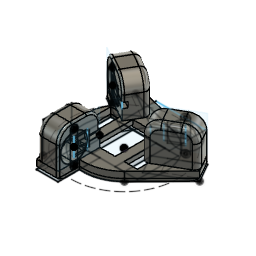
head (Autodesk Fusion 360 design; units mm, degrees)
Autodesk Fusion 360 part; units mm, degrees
note: some values were not read from the file. Set by a fixed rule: which sketch regions a step uses.
sketch "Sketch1" plane through (0, 0, 0) normal (0, 1, 0) x (1, 0, 0)
  line L0 (-38, 23) -> (38, 23)
  line L1 (38, 23) -> (38, -23)
  line L2 (38, -23) -> (-38, -23)
  line L3 (-38, -23) -> (-38, 23)
  line L4 (-28, 23) -> (28, 23)
  line L5 (28, 23) -> (28, 63.9462)
  line L6 (28, 63.9462) -> (-28, 63.9462)
  line L7 (-28, 63.9462) -> (-28, 23)
  circle A0 centre (0, 0) radius 60 construction
  line L8 (-4.5, -70) -> (-28.5, -70)
  line L9 (-28.5, -70) -> (-28.5, -23)
  line L10 (-28.5, -23) -> (-4.5, -23)
  line L11 (-4.5, -23) -> (-4.5, -70)
  line L12 (-4.5, -67) -> (-24.5, -67) construction
  line L13 (-24.5, -67) -> (-24.5, -37) construction
  line L14 (-24.5, -37) -> (-4.5, -37) construction
  line L15 (-4.5, -37) -> (-4.5, -67) construction
  line L16 (34.1686, -13.1817) -> (22.1686, 7.6029)
  line L17 (74.8718, 10.3183) -> (34.1686, -13.1817)
  line L18 (22.1686, 7.6029) -> (62.8718, 31.1029)
  line L19 (62.8718, 31.1029) -> (74.8718, 10.3183)
  line L20 (70.2737, 12.2824) -> (44.2929, -2.7176) construction
  line L21 (44.2929, -2.7176) -> (34.2929, 14.6029) construction
  line L22 (60.2737, 29.6029) -> (70.2737, 12.2824) construction
  line L23 (34.2929, 14.6029) -> (60.2737, 29.6029) construction
  line L24 (-5.6686, 36.1817) -> (-17.6686, 15.3971)
  line L25 (-46.3718, 59.6817) -> (-5.6686, 36.1817)
  line L26 (-17.6686, 15.3971) -> (-58.3718, 38.8971)
  line L27 (-58.3718, 38.8971) -> (-46.3718, 59.6817)
  line L28 (-45.7737, 54.7176) -> (-19.7929, 39.7176) construction
  line L29 (-19.7929, 39.7176) -> (-29.7929, 22.3971) construction
  line L30 (-55.7737, 37.3971) -> (-45.7737, 54.7176) construction
  line L31 (-29.7929, 22.3971) -> (-55.7737, 37.3971) construction
  circle A1 centre (0, 0) radius 46
  line L32 (-28.5, -70) -> (-44.3617, -12.167)
  line L33 (74.8718, 10.3183) -> (32.7178, -32.3349)
  line L34 (-46.3718, 59.6817) -> (11.6439, 44.5019)
  line L35 (-23, -23) -> (-13, -23)
  line L36 (-13, -23) -> (-13, 23)
  line L37 (-13, 23) -> (-23, 23)
  line L38 (-23, 23) -> (-23, -23)
  line L39 (13, -23) -> (23, -23)
  line L40 (23, -23) -> (23, 23)
  line L41 (23, 23) -> (13, 23)
  line L42 (13, 23) -> (13, -23)
  dimension "d1" = 76
  dimension "d2" = 38
  dimension "d3" = 46
  dimension "d4" = 23
  dimension "d5" = 56
  dimension "d6" = 28
  dimension "d7" = 120
  dimension "d8" = 24
  dimension "d9" = 4.5
  dimension "d10" = 70
  dimension "d11" = 20
  dimension "d12" = 30
  dimension "d13" = 67
  dimension "d15" = 360
  dimension "d16" = 92
  dimension "d18" = 360
  dimension "d24" = 15
  dimension "d25" = 10
  dimension "d26" = 10
  dimension "d27" = 15
  constraint horizontal L0
  constraint vertical L1
  constraint horizontal L2
  constraint vertical L3
  constraint horizontal L4
  constraint vertical L5
  constraint horizontal L6
  constraint vertical L7
  constraint coincident L0 L4.start
  constraint coincident A0.centre A1.centre
  constraint horizontal L8
  constraint vertical L9
  constraint horizontal L10
  constraint vertical L11
  constraint coincident L2 L9.end
  constraint horizontal L12
  constraint vertical L13
  constraint horizontal L14
  constraint vertical L15
  constraint coincident L11 L12.start
  constraint concentric A0 A1
  constraint coincident A1 L32.end
  constraint tangent A1 L32
  constraint horizontal L35
  constraint vertical L36
  constraint horizontal L37
  constraint vertical L38
  constraint coincident L0 L36.end
  constraint coincident L10 L35.start
  constraint horizontal L39
  constraint vertical L40
  constraint horizontal L41
  constraint vertical L42
  constraint coincident L0 L40.end
  constraint coincident L2 L39.start
  measures "d1" distance of L0.start L0.end
  measures "d2" distance of A0.centre L3
  measures "d3" distance of L0.start L2.end
  measures "d4" distance of A0.centre L0
  measures "d5" distance of L5.end L6.end
  measures "d6" distance of A0.centre L7
  measures "d7" diameter of A0
  measures "d8" distance of L8.start L8.end
  measures "d9" distance of A0.centre L11
  measures "d10" distance of A0.centre L8
  measures "d11" distance of L12.start L12.end
  measures "d12" distance of L12.start L14.end
  measures "d13" distance of A0.centre L12
  measures "d16" diameter of A1
  measures "d24" distance of L3 L38
  measures "d25" distance of L36 L38
  measures "d26" distance of L40 L42
  measures "d27" distance of L1 L40
extrude "Extrude1" add sketch "Sketch1" along normal blind 3 contours L0 L7 L26 A1 | L0 L2 L3 L9 L26 A1 | L7 L25 L26 L27 A1 | L2 L9 L10 L11 A1 L35 | L9 A1 L32 | L8 L9 L11 A1 | L0 L1 L5 L18 A1 | L1 L2 L11 L17 A1 L39 | L17 L18 L19 A1 | L17 A1 L33 makes body 1 at (-23.6667, 0, 46.2598)
extrude "Extrude2" add sketch "Sketch1" along normal blind 2 from surface at 3 separate body contours L0 L4 L7 L24 L25 A1 L37 | L0 L7 L26 A1 | L0 L2 L3 L9 L26 A1 | L7 L25 L26 L27 A1 | L7 L25 A1 | L0 L4 L5 L24 L25 A1 L37 L41 | L7 L25 L34 | L7 L25 A1 L34 | L2 L9 L10 L11 A1 L35 | L9 A1 L32 | L8 L9 L11 A1 | L0 L1 L5 L18 A1 | L1 L2 L11 L17 A1 L39 | L1 L17 L18 A1 | L17 L18 L19 A1 | L17 A1 L33 makes body 2
extrude "Extrude3" add sketch "Sketch1" along normal blind 5 from surface at 5 contours L0 L4 L7 L24 L25 A1 L37 | L0 L7 L26 A1 | L0 L4 L24 L26 L37 L38 | L0 L2 L3 L9 L26 A1 | L7 L25 L26 L27 A1 | L7 L25 A1 | L0 L4 L5 L24 L25 A1 L37 L41 | L0 L2 L4 L10 L24 L26 L35 L36 L37 L38 | L7 L25 L34 | L7 L25 A1 L34 | L2 L9 L10 L11 A1 L35 | L9 A1 L32 | L0 L2 L4 L16 L18 L39 L40 L41 L42 | L8 L9 L11 A1 | L0 L1 L5 L18 A1 | L1 L2 L11 L17 A1 L39 | L1 L17 L18 A1 | L17 L18 L19 A1 | L17 A1 L33 bodies 2
extrude "Extrude4" add sketch "Sketch1" along normal blind 40 from surface at 10 separate body contours L0 L4 L7 L24 L25 A1 L37 | L0 L4 L26 L38 | L0 L7 L26 A1 | L0 L4 L24 L26 L37 L38 | L7 L25 L26 L27 A1 | L7 L25 A1 | L2 L9 L10 L11 A1 L35 | L8 L9 L11 A1 | L1 L17 L18 A1 | L17 L18 L19 A1 | L16 L18 L40 | L1 L16 L17 L18 L40 makes body 3 at (61.304, 36.6667, -2.4849) makes body 4 at (-4.5, 36.6667, 38.6667) makes body 5 at (-32.804, 36.6667, -51.8484)
sketch "Sketch2" plane through (-4.5, 0, 0) normal (1, 0, 0) x (0, 0, -1)
  line L0 (-70, 10) -> (-23, 10)
  line L1 (-23, 10) -> (-23, 50)
  line L2 (-23, 50) -> (-70, 50)
  line L3 (-70, 50) -> (-70, 10)
  circle A0 centre (-52, 25) radius 15
  circle A1 centre (-52, 42.75) radius 4
  circle A2 centre (-52, 7.25) radius 4
  line L4 (-56, 42.75) -> (-56, 7.25)
  line L5 (-48, 42.75) -> (-48, 7.25)
  line L6 (-52, 33) -> (-35, 33)
  line L7 (-35, 33) -> (-35, 17)
  line L8 (-35, 17) -> (-52, 17)
  line L9 (-52, 17) -> (-52, 33)
  line L10 (-52, 28) -> (-23, 28)
  line L11 (-23, 28) -> (-23, 22)
  line L12 (-23, 22) -> (-52, 22)
  line L13 (-52, 22) -> (-52, 28)
  circle A3 centre (-52, 42.75) radius 1.3
  circle A4 centre (-52, 7.25) radius 1.3
  line L14 (-52, 35) -> (-37, 35)
  line L15 (-37, 35) -> (-37, 15)
  line L16 (-37, 15) -> (-52, 15)
  line L17 (-52, 15) -> (-52, 35)
  dimension "d34" = 30
  dimension "d35" = 18
  dimension "d36" = 8
  dimension "d37" = 8
  dimension "d38" = 35.5
  dimension "d39" = 17.75
  dimension "d40" = 16
  dimension "d41" = 8
  dimension "d42" = 17
  dimension "d43" = 6
  dimension "d44" = 3
  dimension "d45" = 2.6
  dimension "d46" = 2.6
  dimension "d47" = 20
  dimension "d48" = 10
  constraint vertical A0.centre A1.centre
  constraint vertical A0.centre A2.centre
  constraint tangent L0 A0
  constraint coincident A1 L4.start
  constraint coincident A2 L4.end
  constraint tangent A2 L4
  constraint coincident A1 L5.start
  constraint coincident A2 L5.end
  constraint perpendicular L0 L5
  constraint tangent A1 L5
  constraint tangent A1 L4
  constraint horizontal L6
  constraint vertical L7
  constraint horizontal L8
  constraint vertical L9
  constraint coincident A0.centre L9
  constraint horizontal L10
  constraint vertical L11
  constraint horizontal L12
  constraint vertical L13
  constraint coincident L1 L11.end
  constraint coincident L9 L10.start
  constraint concentric A1 A3
  constraint concentric A2 A4
  constraint horizontal L14
  constraint vertical L15
  constraint horizontal L16
  constraint vertical L17
  measures "d34" diameter of A0
  measures "d35" distance of L3 A0.centre
  measures "d36" diameter of A1
  measures "d37" diameter of A2
  measures "d38" distance of A1.centre A2.centre
  measures "d39" distance of A0.centre A2.centre
  measures "d40" distance of L6.end L7.end
  measures "d41" distance of A0.centre L8
  measures "d42" distance of A0.centre L7
  measures "d43" distance of L10.end L11.end
  measures "d44" distance of A0.centre L10
  measures "d45" diameter of A3
  measures "d46" diameter of A4
  measures "d47" distance of L14.end L15.end
  measures "d48" distance of A0.centre L14
extrude "Extrude5" cut sketch "Sketch2" against normal blind 20 contours A0 A1 A2 L4 L5 L9 L13 L14 L16 L17 | A0 L4 | A0 A2 | A0 A1 | L6 L7 L10 L15 | L7 L10 L12 L15 | A0 L5 L16 | L7 L8 L12 L15 | A0 L10 L15 | A0 L6 L10 L15 | A0 L5 L8 L16 | A0 L8 L15 L16 | L5 L8 L16 L17 | A0 L5 L14 | A0 L8 L12 L15 | A0 L12 L15 | A0 L6 L14 L15 | A0 L5 L6 L10 | A0 L5 L10 L12 | A0 L5 L8 L12 | L5 L8 L9 L12 L17 | A0 L5 L6 L14 | L5 L6 L14 L17 | L5 L6 L9 L10 L17 | L5 L9 L10 L12 L13 L17 | A3 | A4 picked at (-52, 39.5657) bodies 2 4
extrude "Extrude6" cut sketch "Sketch2" against normal blind 5 contours L1 L7 L10 L11 L12 bodies 4
extrude "Extrude7" cut sketch "Sketch2" against normal blind 1 contours L0 A0 A2 L4 | L0 A2 L4 | L0 A0 A2 | L0 A2 | L0 A0 A2 | A0 A1 L4 | L0 A2 L5 | L0 A0 A2 L5 | A0 A1 | A0 A1 L5 picked at (-53.5011, 40.5339) bodies 2 4
sketch "Sketch3" plane through (2.25, 0, -3.8971) normal (-0.5, 0, 0.866025) x (0.866025, 0, 0.5)
  line L0 (-70, 10) -> (-23, 10)
  line L1 (-23, 10) -> (-23, 50)
  line L2 (-23, 50) -> (-70, 50)
  line L3 (-70, 50) -> (-70, 10)
  circle A0 centre (-52, 25) radius 15
  circle A1 centre (-52, 42.75) radius 4
  circle A2 centre (-52, 7.25) radius 4
  line L4 (-52, 35) -> (-37, 35)
  line L5 (-37, 35) -> (-37, 15)
  line L6 (-37, 15) -> (-52, 15)
  line L7 (-52, 15) -> (-52, 35)
  line L8 (-52, 33) -> (-35, 33)
  line L9 (-35, 33) -> (-35, 17)
  line L10 (-35, 17) -> (-52, 17)
  line L11 (-52, 17) -> (-52, 33)
  line L12 (-52, 28) -> (-23, 28)
  line L13 (-23, 28) -> (-23, 22)
  line L14 (-23, 22) -> (-52, 22)
  line L15 (-52, 22) -> (-52, 28)
  line L16 (-56, 42.75) -> (-56, 7.25)
  line L17 (-48, 7.25) -> (-48, 42.75)
  circle A3 centre (-52, 42.75) radius 1.3
  circle A4 centre (-52, 7.25) radius 1.3
  dimension "d55" = 30
  dimension "d56" = 8
  dimension "d57" = 8
  dimension "d58" = 18
  dimension "d59" = 35.5
  dimension "d60" = 17.75
  dimension "d61" = 6
  dimension "d62" = 16
  dimension "d63" = 20
  dimension "d64" = 10
  dimension "d65" = 8
  dimension "d66" = 3
  dimension "d67" = 17
  dimension "d68" = 2.6
  dimension "d69" = 2.6
  constraint vertical A0.centre A2.centre
  constraint vertical A0.centre A1.centre
  constraint tangent L0 A0
  constraint horizontal L4
  constraint vertical L5
  constraint horizontal L6
  constraint vertical L7
  constraint horizontal L8
  constraint vertical L9
  constraint horizontal L10
  constraint vertical L11
  constraint coincident L7 L8.start
  constraint horizontal L12
  constraint vertical L13
  constraint horizontal L14
  constraint vertical L15
  constraint coincident L7 L12.start
  constraint tangent A0 L5
  constraint coincident A0.centre L7
  constraint coincident A1 L16.start
  constraint coincident A2 L16.end
  constraint perpendicular L0 L16
  constraint coincident A2 L17.start
  constraint coincident A1 L17.end
  constraint tangent A1 L17
  constraint tangent A1 L16
  constraint tangent A2 L17
  constraint concentric A1 A3
  constraint concentric A2 A4
  measures "d55" diameter of A0
  measures "d56" diameter of A1
  measures "d57" diameter of A2
  measures "d58" distance of L3 A0.centre
  measures "d59" distance of A1.centre A2.centre
  measures "d60" distance of A0.centre A2.centre
  measures "d61" distance of L12.end L13.end
  measures "d62" distance of L8.end L9.end
  measures "d63" distance of L4.end L5.end
  measures "d64" distance of A0.centre L4
  measures "d65" distance of A0.centre L8
  measures "d66" distance of A0.centre L12
  measures "d67" distance of L8.start L8.end
  measures "d68" diameter of A3
  measures "d69" diameter of A4
extrude "Extrude8" cut sketch "Sketch3" against normal blind 20 contours A0 A1 A2 L4 L6 L7 L11 L15 L16 L17 | A0 L16 | A0 A2 | A0 A1 | L5 L8 L9 L12 | L5 L9 L12 L14 | A0 L6 L17 | L5 L9 L10 L14 | A0 L5 L8 L12 | A0 L5 L12 | A0 L6 L10 L17 | A0 L5 L6 L10 | L6 L7 L10 L17 | A0 L4 L17 | A0 L5 L14 | A0 L5 L10 L14 | A0 L4 L5 L8 | A0 L12 L14 L17 | A0 L8 L12 L17 | A0 L10 L14 L17 | L7 L10 L11 L14 L17 | A0 L4 L8 L17 | L4 L7 L8 L17 | L7 L11 L12 L14 L15 L17 | L7 L8 L11 L12 L17 | A3 | A4 picked at (-52, 39.5657) bodies 2 5
extrude "Extrude9" cut sketch "Sketch3" against normal blind 5 contours L1 L9 L12 L13 L14 bodies 5
extrude "Extrude10" cut sketch "Sketch3" against normal blind 1 contours L0 A0 A2 L16 | L0 A2 L16 | L0 A0 A2 | L0 A2 | L0 A0 A2 | A0 A1 L16 | L0 A2 L17 | L0 A0 A2 L17 | A0 A1 | A0 A1 L17 picked at (-50.4989, 40.5339) bodies 2 5
sketch "Sketch4" plane through (2.25, 0, 3.8971) normal (-0.5, 0, -0.866025) x (-0.866025, 0, 0.5)
  line L0 (-70, 10) -> (-23, 10)
  line L1 (-23, 10) -> (-23, 50)
  line L2 (-23, 50) -> (-70, 50)
  line L3 (-70, 50) -> (-70, 10)
  circle A0 centre (-52, 25) radius 15
  circle A1 centre (-52, 42.75) radius 4
  circle A2 centre (-52, 7.25) radius 4
  circle A3 centre (-52, 42.75) radius 1.3
  circle A4 centre (-52, 7.25) radius 1.3
  line L4 (-56, 7.25) -> (-56, 42.75)
  line L5 (-48, 42.75) -> (-48, 7.25)
  line L6 (-52, 35) -> (-37, 35)
  line L7 (-37, 35) -> (-37, 15)
  line L8 (-37, 15) -> (-52, 15)
  line L9 (-52, 15) -> (-52, 35)
  line L10 (-52, 33) -> (-34, 33)
  line L11 (-34, 33) -> (-34, 17)
  line L12 (-34, 17) -> (-52, 17)
  line L13 (-52, 17) -> (-52, 33)
  line L14 (-52, 28) -> (-23, 28)
  line L15 (-23, 28) -> (-23, 22)
  line L16 (-23, 22) -> (-52, 22)
  line L17 (-52, 22) -> (-52, 28)
  dimension "d76" = 30
  dimension "d77" = 8
  dimension "d78" = 8
  dimension "d79" = 17.75
  dimension "d80" = 35.5
  dimension "d81" = 18
  dimension "d82" = 2.6
  dimension "d83" = 2.6
  dimension "d84" = 20
  dimension "d85" = 10
  dimension "d86" = 16
  dimension "d87" = 8
  dimension "d88" = 3
  dimension "d89" = 6
  constraint vertical A0.centre A2.centre
  constraint vertical A0.centre A1.centre
  constraint concentric A1 A3
  constraint concentric A2 A4
  constraint tangent L0 A0
  constraint coincident A2 L4.start
  constraint coincident A1 L4.end
  constraint tangent A1 L4
  constraint coincident A1 L5.start
  constraint coincident A2 L5.end
  constraint tangent A2 L5
  constraint tangent A2 L4
  constraint tangent A1 L5
  constraint horizontal L6
  constraint vertical L7
  constraint horizontal L8
  constraint vertical L9
  constraint tangent A0 L7
  constraint horizontal L10
  constraint vertical L11
  constraint horizontal L12
  constraint vertical L13
  constraint coincident L9 L10.start
  constraint horizontal L14
  constraint vertical L15
  constraint horizontal L16
  constraint vertical L17
  constraint coincident L9 L14.start
  measures "d76" diameter of A0
  measures "d77" diameter of A1
  measures "d78" diameter of A2
  measures "d79" distance of A0.centre A2.centre
  measures "d80" distance of A1.centre A2.centre
  measures "d81" distance of L3 A0.centre
  measures "d82" diameter of A3
  measures "d83" diameter of A4
  measures "d84" distance of L6.end L7.end
  measures "d85" distance of A0.centre L6
  measures "d86" distance of L10.end L11.end
  measures "d87" distance of A0.centre L10
  measures "d88" distance of A0.centre L14
  measures "d89" distance of L14.end L15.end
extrude "Extrude11" cut sketch "Sketch4" against normal blind 20 contours A0 A1 A2 L4 L5 L6 L8 L9 L13 L17 | A0 L4 | A0 A2 | A0 A1 | L7 L10 L11 L14 | L7 L11 L14 L16 | A0 L5 L8 | L7 L11 L12 L16 | A0 L7 L10 L14 | A0 L7 L14 | A0 L5 L8 L12 | A0 L7 L8 L12 | L5 L8 L9 L12 | A0 L5 L6 | A0 L7 L16 | A0 L7 L12 L16 | A0 L6 L7 L10 | A0 L5 L14 L16 | A0 L5 L10 L14 | A0 L5 L12 L16 | L5 L9 L12 L13 L16 | A0 L5 L6 L10 | L5 L6 L9 L10 | L5 L9 L10 L13 L14 | L5 L9 L13 L14 L16 L17 | A3 | A4 picked at (-52, 39.5657) bodies 2 3
extrude "Extrude12" cut sketch "Sketch4" against normal blind 5 contours L1 L11 L14 L15 L16 bodies 3
extrude "Extrude13" cut sketch "Sketch4" against normal blind 1 contours L0 A0 A2 L4 | L0 A2 L4 | L0 A0 A2 | L0 A2 | L0 A0 A2 | L0 A2 L5 | A0 A1 L4 | L0 A0 A2 L5 | A0 A1 | A0 A1 L5 picked at (-50.4989, 40.5339) bodies 2 3
fillet "Fillet1" radius 15 9 edges at (68.8718, 0, -20.7106) (-52.3718, 0, -49.2894) (-16.5, 0, 70) (68.8718, 50, -20.7106) (28.1686, 50, 2.7894) (-16.5, 50, 23) (-16.5, 50, 70) (-52.3718, 50, -49.2894) (-11.6686, 50, -25.7894) on bodies 1 3 4 5
fillet "Fillet2" radius 6 15 edges at (34.1686, 22.5, 13.1817) (37.9734, 45.6066, 10.985) (54.5202, 50, 1.4317) (71.067, 45.6066, -8.1216) (74.8718, 22.5, -10.3183) (-28.5, 22.5, 23) (-28.5, 45.6066, 27.3934) (-28.5, 50, 46.5) (-28.5, 45.6066, 65.6066) (-28.5, 22.5, 70) (-5.6686, 22.5, -36.1817) (-9.4734, 45.6066, -38.3784) (-26.0202, 50, -47.9317) (-42.567, 45.6066, -57.485) (-46.3718, 22.5, -59.6817) on bodies 3 4 5
fillet "Fillet3" radius 2 15 edges at (62.8718, 22.5, -31.1029) (59.067, 45.6066, -28.9062) (42.5202, 50, -19.3529) (25.9734, 45.6066, -9.7996) (22.1686, 31.5, -7.6029) (-4.5, 22.5, 70) (-4.5, 45.6066, 65.6066) (-4.5, 50, 46.5) (-4.5, 45.6066, 27.3934) (-4.5, 31.5, 23) (-58.3718, 22.5, -38.8971) (-54.567, 45.6066, -36.7004) (-38.0202, 50, -27.1471) (-21.4734, 45.6066, -17.5938) (-17.6686, 31.5, -15.3971) on bodies 3 4 5
fillet "Fillet4" radius 2 3 edges at (62.8718, 6.5, -31.1029) (-58.3718, 6.5, -38.8971) (-4.5, 6.5, 70) on bodies 2
sketch "Sketch5" plane through (-28.5, 0, 0) normal (-1, 0, 0) x (0, 0, 1)
  line L0 (64, 10) -> (64, 35)
  arc A0 (64, 35) -> (55, 44) centre (55, 35) ccw
  line L1 (55, 44) -> (38, 44)
  arc A1 (38, 44) -> (29, 35) centre (38, 35) ccw
  line L2 (29, 35) -> (29, 10)
  line L3 (29, 10) -> (64, 10)
  line L4 (30.5, 45) -> (62.5, 45)
  line L5 (62.5, 45) -> (62.5, 10)
  line L6 (62.5, 10) -> (30.5, 10)
  line L7 (30.5, 10) -> (30.5, 45)
  dimension "d104" = 35
  dimension "d105" = 32
  dimension "d106" = 1.5
  constraint horizontal L4
  constraint vertical L5
  constraint horizontal L6
  constraint vertical L7
  constraint coincident L3 L5.end
  measures "d104" distance of L4.start L6.end
  measures "d105" distance of L4.start L4.end
  measures "d106" distance of L2 L7
